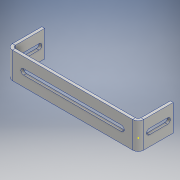
# Autodesk Inventor part: cup
Saved by Autodesk Inventor 2018 (Build 220112000, 112)
## iProperties
Created: 2018-04-05
Part Number: cup
Material: アルミニウム 6061
Document SubType Name: Sheet Metal
Designer: NaMACHAN
Density: 2.7 g/cm^3
Sheet Metal Rule: Default_mm
Appearance: アルミニウム - フラット
Mass: 7.82705 g
Surface Area: 46.2396 cm^2
Volume: 2.89891 cm^3
Flat Pattern Width: 1.9 cm
Flat Pattern Length: 13.7048 cm
Flat Pattern Area: 26.0391 cm^2
Sheet Metal Width: 19.000 mm
Sheet Metal Length: 137.048 mm
Sheet Metal Area: 2603.908 mm^2
Author: NaMACHAN
Autodesk Inventor part; units mm, degrees
ref_plane "YZ Plane" through (0, 0, 0) normal (1, 0, 0) x (0, 1, 0)
ref_plane "XZ Plane" through (0, 0, 0) normal (0, 1, 0) x (-1, 0, 0)
ref_plane "XY Plane" through (0, 0, 0) normal (0, 0, 1) x (1, 0, 0)
sketch "スケッチ1" plane through (0, 0, 0) normal (0, 1, 0) x (-1, 0, 0)
  line L0 (-47, -9.5) -> (47, -9.5)
  line L1 (47, -9.5) -> (47, 9.5)
  line L2 (47, 9.5) -> (-47, 9.5)
  line L3 (-47, 9.5) -> (-47, -9.5)
  line L4 (-47, -9.5) -> (47, 9.5) construction
  line L5 (47, -9.5) -> (-47, 9.5) construction
  point P0 (0, 0)
  dimension "d0" = 94
  dimension "d1" = 19
  measures "d0" distance of L2.end L1.end
  measures "d1" distance of L0.end L1.end
extrude "プレート1" add sketch "スケッチ1" along normal blind 2
sketch "スケッチ2" plane through (45, 0, -9.5) normal (1, 0, 0) x (0, 1, 0)
  line L0 (0, 19) -> (0, 0)
  line L1 (0, 0) -> (25, 0)
  line L2 (25, 0) -> (25, 19)
  line L3 (25, 19) -> (0, 19)
  constraints: 6 end point, 1 horizontal, 1 perpendicular, 1 vertical
edge flange "フランジ1" height 25 angle 90 thickness 2 bend radius 2 thickness toward (1, 0, 0) relief tear relief width 2 relief depth 1 edges at (47, 2, 0) wall of the first edge with corners at (45, 0, 9.5) (45, 0, -9.5) (45, 25, -9.5) (45, 25, 9.5)
bend "曲げ1"
corner "コーナー1"
sketch "スケッチ3" plane through (-45, 0, 9.5) normal (-1, 0, 0) x (0, -1, 0)
  line L0 (0, -19) -> (0, 0)
  line L1 (0, 0) -> (-25, 0)
  line L2 (-25, 0) -> (-25, -19)
  line L3 (-25, -19) -> (0, -19)
  constraints: 6 end point, 1 horizontal, 1 perpendicular, 1 vertical
edge flange "フランジ2" height 25 angle 90 thickness 2 bend radius 2 thickness toward (-1, 0, 0) relief tear relief width 2 relief depth 1 edges at (-47, 2, 0) wall of the first edge with corners at (-45, 0, -9.5) (-45, 0, 9.5) (-45, 25, 9.5) (-45, 25, -9.5)
bend "曲げ2"
corner "コーナー2"
sketch "スケッチ5" plane through (0, 0, 0) normal (0, -1, 0) x (1, 0, 0)
  arc A0 (-35, 2) -> (-35, -2) centre (-35, 0) ccw
  arc A1 (35, -2) -> (35, 2) centre (35, 0) ccw
  line L0 (-35, 2) -> (35, 2)
  line L1 (35, -2) -> (-35, -2)
  point P0 (0, 0)
  dimension "d31" = 4
  dimension "d32" = 2
  dimension "d33" = 2
  dimension "d34" = 2
  dimension "d35" = 35
  dimension "d36" = 35
  constraints: 4 end point, 4 point on circle, 2 centre point, 2 horizontal, 2 vertical alignment
  measures "d31" distance between parallel lines of L0 L1
  measures "d32" radius of A1
  measures "d33" radius of A0
  measures "d34" distance from line of L0 point (0, 0)
  measures "d35" distance of point (0, 0) A0.centre
  measures "d36" distance of A1.centre point (0, 0)
extrude "押し出し1" cut sketch "スケッチ5" against normal blind 2
sketch "スケッチ6" plane through (47, 25, 9.5) normal (1, 0, 0) x (0, 0, -1)
  point P0 (9.5, -25)
sketch "スケッチ7" plane through (47, 25, 9.5) normal (1, 0, 0) x (0, 0, -1)
  line L0 (7.5, -4) -> (7.5, -17)
  arc A0 (7.5, -17) -> (11.5, -17) centre (9.5, -17) ccw
  line L1 (11.5, -17) -> (11.5, -4)
  arc A1 (11.5, -4) -> (7.5, -4) centre (9.5, -4) ccw
  line L2 (0, 0) -> (19, 0) projected
  line L3 (0, -21) -> (19, -21) projected
  point P0 (9.5, -25)
  point P1 (9.5, 0)
  dimension "d45" = 4
  dimension "d46" = 4
  dimension "d47" = 2
  constraints: 4 end point, 4 point on circle, 4 tangent, 2 centre point, 1 midpoint, 1 parallel, 1 vertical, 1 vertical alignment
  measures "d45" distance from line of L2 A1.centre
  measures "d46" distance from line of L3 A0.centre
  measures "d47" radius of A1
extrude "押し出し2" cut sketch "スケッチ7" against normal blind 100
equation "\"d2\" = Thickness"
equation "\"d3\" = BendReliefWidth"
equation "\"d4\" = BendReliefDepth"
equation "\"d5\" = MinimumRemnant"
equation "\"d6\" = TransitionRadius"
equation "\"d9\" = BendRadius"
equation "\"d10\" = CornerReliefSize"
equation "\"d11\" = GapSize"
equation "\"d12\" = JacobiRadiusSize"
equation "\"d13\" = BendReliefWidth"
equation "\"d14\" = BendReliefDepth"
equation "\"d15\" = MinimumRemnant"
equation "\"d16\" = TransitionRadius"
equation "\"d19\" = BendRadius"
equation "\"d20\" = CornerReliefSize"
equation "\"d21\" = GapSize"
equation "\"d22\" = JacobiRadiusSize"
equation "\"BendRadius\" = Thickness"
equation "\"BendReliefWidth\" = Thickness"
equation "\"BendReliefDepth\" = 0.5 * Thickness"
equation "\"CornerReliefSize\" = 4 * Thickness"
equation "\"MinimumRemnant\" = 2 * Thickness"
equation "\"TransitionRadius\" = BendRadius"
equation "\"JacobiRadiusSize\" = BendRadius"
equation "\"GapSize\" = Thickness"
equation "\"Thickness\" = 2"
